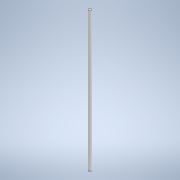
# Autodesk Inventor part: rail_300
Saved by Autodesk Inventor 2021 (Build 250183000, 183)
## iProperties
Created: 2023-01-31
Part Number: rail_300
Material: Типовые
Document SubType Name: Modeling
Designer: ignat
Density: 1 g/cm^3
Appearance: По умолчанию
Author: ignat
Autodesk Inventor part; units mm, degrees
ref_plane "YZ Plane" through (0, 0, 0) normal (1, 0, 0) x (0, 1, 0)
ref_plane "XZ Plane" through (0, 0, 0) normal (0, 1, 0) x (-1, 0, 0)
ref_plane "XY Plane" through (0, 0, 0) normal (0, 0, 1) x (1, 0, 0)
sketch "Эскиз1" plane through (0, 0, 0) normal (0, 1, 0) x (-1, 0, 0)
  circle A0 centre (0, 0) radius 4
  dimension "d0" = 8
  constraints: 1 centre point, 1 coincident
  measures "d0" diameter of A0
extrude "Выдавливание1" add sketch "Эскиз1" along normal mid plane 400
